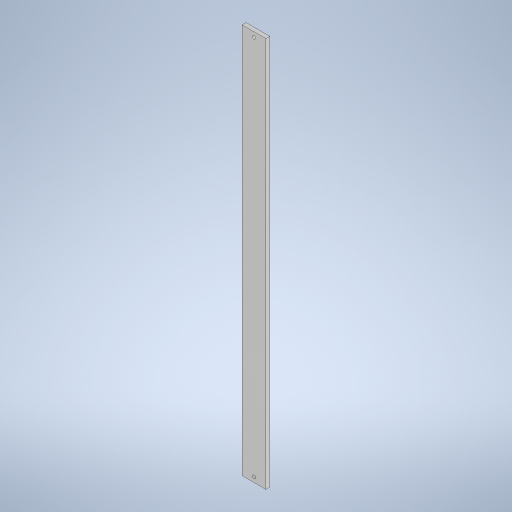
# Autodesk Inventor part: Barra le
Saved by Autodesk Inventor 2023.2 (Build 272271030, 271C)
## iProperties
Created: 2023-03-21
Part Number: Barra le
Material: Alumínio 6061
Document SubType Name: Sheet Metal
Designer: Mateus
Density: 2.7 g/cm^3
Sheet Metal Rule: Padrão_mm
Appearance: Usinado - Alumínio
Mass: 200.07 g
Surface Area: 348.8 cm^2
Volume: 74.1 cm^3
Author: Mateus
Autodesk Inventor part; units mm, degrees
ref_plane "YZ Plane" through (0, 0, 0) normal (1, 0, 0) x (0, 1, 0)
ref_plane "XZ Plane" through (0, 0, 0) normal (0, 1, 0) x (-1, 0, 0)
ref_plane "XY Plane" through (0, 0, 0) normal (0, 0, 1) x (1, 0, 0)
sketch "Esboço1" plane through (0, 0, 0) normal (0, 1, 0) x (-1, 0, 0)
  line L0 (0, 0) -> (30, 0)
  line L1 (30, 0) -> (30, -5)
  line L2 (30, -5) -> (0, -5)
  line L3 (0, -5) -> (0, 0)
  dimension "d0" = 30
  dimension "d1" = 5
  constraints: 8 end point, 2 parallel, 1 horizontal, 1 perpendicular
  measures "d0" distance of L1.end L2.end
  measures "d1" distance of L2.end L0.start
extrude "Extrusão1" add sketch "Esboço1" along normal blind 494
sketch "Esboço4" plane through (-30, 0, 0) normal (0, 0, 1) x (1, 0, 0)
  line L0 (0, 494) -> (30, 494) projected
  line L1 (30, 0) -> (30, 494) projected
  line L2 (0, 0) -> (30, 0) projected
  point P0 (15, 6.25)
  point P1 (15, 487.75)
  dimension "d30" = 30
  dimension "d31" = 15
  dimension "d32" = 15
  dimension "d33" = 6.25
  dimension "d34" = 6.25
  measures "d30" distance of L0.start L0.end
  measures "d31" distance from line of point (15, 487.75) L1
  measures "d32" distance from line of L1 point (15, 6.25)
  measures "d33" distance from line of L0 point (15, 487.75)
  measures "d34" distance from line of L2 point (15, 6.25)
hole "Furo3" at (-15, 487.75, 0) at (-15, 6.25, 0) direction (0, 0, -1) diameter 4 end through all
equation "\"d31\" = 0.5 * d30"
equation "\"d32\" = d31"
equation "\"d34\" = d33"
equation "\"d40\" = Espessura"
equation "\"Raio_vergadura\" = Espessura"
equation "\"Largura_alívio_de_vergadura\" = Espessura"
equation "\"Profundidade_alívio_de_vergadura\" = 0.5 * Espessura"
equation "\"Tamanho_alívio_de_dobra\" = 4 * Espessura"
equation "\"Remanescente_mínimo\" = 2 * Espessura"
equation "\"Raiodetransição\" = Raio_vergadura"
equation "\"Tamanho_de_raio_de_Jacobi\" = Raio_vergadura"
equation "\"TamanhoFolga\" = Espessura"
equation "\"Espessura\" = 0.5"
